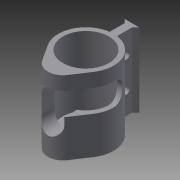
# Autodesk Inventor part: bikeLockMountV2part1
Saved by Autodesk Inventor 2015 (Build 190159000, 159)
## iProperties
Created: 2015-01-18
Part Number: bikeLockMountV2part1
Material: Generic
Document SubType Name: Modeling
Designer: rmsin_000
Density: 1 g/cm^3
Appearance: Default
Author: rmsin_000
Autodesk Inventor part; units mm, degrees
ref_plane "YZ Plane" through (0, 0, 0) normal (1, 0, 0) x (0, 1, 0)
ref_plane "XZ Plane" through (0, 0, 0) normal (0, 1, 0) x (-1, 0, 0)
ref_plane "XY Plane" through (0, 0, 0) normal (0, 0, 1) x (1, 0, 0)
sketch "Sketch1" plane through (0, 0, 0) normal (0, 1, 0) x (-1, 0, 0)
  line L0 (0, 0) -> (0, 28.1143)
  line L1 (16.7843, 9.0105) -> (8.6989, 21.4436)
  line L2 (-8.6989, 21.4436) -> (-15.9171, 10.4666)
  arc A0 (-15.9171, 10.4666) -> (15.0435, 11.6875) centre (0, 0) ccw
  arc A1 (8.6989, 21.4436) -> (-8.6989, 21.4436) centre (0, 15.7866) ccw
  constraints: 6 end point, 5 point on circle, 2 centre point, 2 point on line, 2 tangent, 1 coincident, 1 vertical
extrude "Extrusion1" add sketch "Sketch1" along normal blind 50.8 contours A0 L2 A1 L1
sketch "Sketch2" plane through (0, 50.8, 0) normal (0, 1, 0) x (1, 0, 0)
  circle A0 centre (0, 0) radius 15.875
  dimension "d3" = 31.75
  constraints: 1 centre point, 1 coincident
  measures "d3" diameter of A0
extrude "Extrusion2" cut sketch "Sketch2" against normal blind 47.625
sketch "Sketch3" plane through (0, 0, 0) normal (0, 0, 1) x (1, 0, 0)
  line L0 (0, 0) -> (0, 12.7)
  line L1 (-7.7476, 33.5742) -> (-7.7472, 20.4468)
  line L2 (7.7474, 33.5741) -> (7.7474, 33.574)
  line L3 (7.747, 25.8264) -> (7.7468, 20.4467)
  line L4 (7.7473, 41.3219) -> (-0.0002, 41.3219)
  arc A0 (0, 41.3219) -> (-7.7476, 33.5742) centre (-0.0001, 33.5744) ccw
  arc A1 (-7.7472, 20.4468) -> (7.7468, 20.4467) centre (-0.0002, 20.447) ccw
  arc A2 (7.747, 25.8264) -> (7.7473, 41.3219) centre (7.7474, 33.5741) ccw
  dimension "d6" = 12.7
  constraints: 10 end point, 8 point on circle, 4 tangent, 3 centre point, 1 coincident, 1 horizontal, 1 point on line, 1 vertical
  measures "d6" distance of L0.start L0.end
extrude "Extrusion3" cut sketch "Sketch3" along normal blind 44.45
sketch "Sketch4" plane through (0, 0, 0) normal (1, 0, 0) x (0, 1, 0)
  arc A0 (25.8264, -0.0001) -> (41.32, -0.0702) centre (33.573, -0.0696) ccw
  line L0 (41.32, -0.0702) -> (41.32, 29.3277)
  line L1 (41.32, 29.3277) -> (25.8264, 29.047)
  line L2 (25.8264, 29.047) -> (25.8264, -0.0001)
  point P0 (0, 0)
  point P1 (25.8264, 17.4036)
  constraints: 6 end point, 2 point on circle, 1 centre point, 1 parallel, 1 vertical
extrude "Extrusion4" cut sketch "Sketch4" along normal blind 44.45
sketch "Sketch5" plane through (0, 0, 0) normal (0, -1, 0) x (1, 0, 0)
  arc A0 (-16.7843, 9.0105) -> (15.9171, 10.4666) centre (0, 0) ccw projected
  line L0 (0, -19.05) -> (0, -31.75)
  line L1 (2.54, -18.8799) -> (2.54, -29.21)
  line L2 (-2.54, -18.8799) -> (-2.54, -29.21)
  line L3 (5.08, -31.75) -> (2.54, -29.21)
  line L4 (-5.08, -31.75) -> (-2.54, -29.21)
  line L5 (5.08, -31.75) -> (-5.08, -31.75)
  arc A1 (-2.54, -18.8799) -> (2.54, -18.8799) centre (0, 0.0817) ccw
  dimension "d13" = 12.7
  dimension "d14" = 5.08
  dimension "d27" = 10.16
  constraints: 12 end point, 4 point on circle, 3 symmetric about line, 3 vertical, 1 centre point, 1 horizontal
  measures "d13" distance of L0.start L0.end
  measures "d14" diameter of L1 L0
  measures "d27" distance of L3.start L4.start
extrude "Extrusion5" add sketch "Sketch5" against normal blind 50.8
sketch "Sketch6" plane through (0, 0, 0) normal (1, 0, 0) x (0, 1, 0)
  line L0 (0, -31.75) -> (50.8, -31.75) projected
  circle A0 centre (35.814, -25.2921) radius 2.286
  circle A1 centre (14.986, -25.2921) radius 2.286
  line L1 (0, -25.2921) -> (12.7, -25.2921)
  line L2 (38.1, -25.2921) -> (50.8, -25.2921)
  line L3 (50.8, -19.05) -> (50.8, 10.4666) projected
  point P0 (0, 0)
  point P1 (50.8, 9.0105)
  dimension "d19" = 4.572
  dimension "d20" = 4.572
  dimension "d23" = 12.7
  dimension "d24" = 12.7
  constraints: 4 end point, 2 horizontal alignment, 1 perpendicular, 5 other
  measures "d23" distance of L1.start L1.end
  measures "d24" distance of L2.start L2.end
extrude "Extrusion6" cut sketch "Sketch6" along normal mid plane 44.45
body "Solid1"
